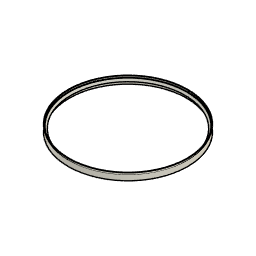
ringclock_outer_ring (Autodesk Fusion 360 design; units mm, degrees)
Autodesk Fusion 360 part; units mm, degrees
note: some values were not read from the file. Set by a fixed rule: which sketch regions a step uses.
sketch "Skizze1" plane through (0, 0, 0) normal (1, 0, 0) x (0, 1, 0)
  line L0 (-111.5, 0) -> (-111.5, 10)
  line L1 (-110.5, 10) -> (-109.5, 10)
  line L2 (-111.5, 0) -> (-109.5, 0)
  line L3 (-109.5, 0) -> (-106.5, 6)
  line L4 (-106.5, 6) -> (-109.5, 10)
  line L5 (0, 0) -> (0, 38) construction
  line L6 (-110.5, 10) -> (-110.5, 13)
  line L7 (-110.5, 13) -> (-111.5, 13)
  line L8 (-111.5, 13) -> (-111.5, 10)
  dimension "d2" = 2
  dimension "d3" = 2
  dimension "d4" = 6
  dimension "d5" = 5
  dimension "d6" = 111.5
  dimension "d9" = 3
  dimension "d10" = 1
  dimension "d11" = 10
  constraint vertical L0
  constraint perpendicular L0 L1
  constraint perpendicular L0 L2
  constraint coincident L5.start L2
  constraint coincident L5.start origin
  constraint vertical L5
  constraint perpendicular L1 L6
  constraint perpendicular L6 L7
  measures "d2" distance of L0.start L2.end
  measures "d3" distance of L0.end L1.end
  measures "d4" vertical distance of L0.start L3.end
  measures "d5" distance of L0 L3.end
  measures "d6" distance of L5.start L0
  measures "d9" distance of L0.end L7.end
  measures "d10" distance of L6 L8
  measures "d11" distance of L0.start L1
revolve "Drehen1" add sketch "Skizze1" angle 360 about axis through (0, 0, 0) along (0, 0, 1)
